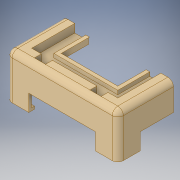
# Autodesk Inventor part: model for case_back
Saved by Autodesk Inventor 2016 (Build 200138000, 138)
## iProperties
Created: 2016-08-06
Part Number: model for case_back
Material: Polyethylene, High Density
Document SubType Name: Modeling
Designer: Jorian Brusind
Density: 0.952 g/cm^3
Appearance: Smooth - Off-White
Author: Jorian Brusind
Autodesk Inventor part; units mm, degrees
ref_plane "YZ Plane" through (0, 0, 0) normal (1, 0, 0) x (0, 1, 0)
ref_plane "XZ Plane" through (0, 0, 0) normal (0, 1, 0) x (-1, 0, 0)
ref_plane "XY Plane" through (0, 0, 0) normal (0, 0, 1) x (1, 0, 0)
sketch "Sketch4" plane through (0, 0, 0) normal (0, 1, 0) x (-1, 0, 0)
  line L0 (0, 0) -> (127, 0)
  line L1 (127, 0) -> (127, -127)
  line L2 (127, -127) -> (0, -127)
  line L3 (0, -127) -> (0, 0)
  dimension "d16" = 127
  dimension "d17" = 127
  constraints: 8 end point, 2 parallel, 1 horizontal, 1 perpendicular
  measures "d16" distance of L1.end L2.end
  measures "d17" distance of L0.end L1.end
extrude "Extrusion4" add sketch "Sketch4" along normal blind 50.8
sketch "Sketch5" plane through (0, 50.8, 0) normal (0, 1, 0) x (1, 0, 0)
  line L0 (0, 0) -> (0, 127) projected
  line L1 (-127, 127) -> (-127, 0) projected
  line L2 (-127, 0) -> (0, 0) projected
  line L3 (0, 127) -> (-127, 127) projected
  line L4 (0, 127) -> (0, 114.3)
  line L5 (-127, 0) -> (-127, 14.2875)
  line L6 (-112.6998, 14.2875) -> (-14.2748, 14.2875)
  line L7 (-14.2748, 14.2875) -> (-14.2748, 112.7125)
  line L8 (-14.2748, 112.7125) -> (-112.6998, 112.7125)
  line L9 (-112.6998, 112.7125) -> (-112.6998, 14.2875)
  line L10 (-112.6998, 14.2875) -> (-112.6998, 26.9875)
  line L11 (-99.9998, 26.9875) -> (-26.9748, 26.9875)
  line L12 (-14.2748, 14.2875) -> (-26.9748, 14.2875)
  line L13 (-26.9748, 26.9875) -> (-26.9748, 100.0125)
  line L14 (-112.6998, 112.7125) -> (-99.9998, 112.7125)
  line L15 (-99.9998, 100.0125) -> (-99.9998, 26.9875)
  line L16 (-112.6998, 112.7125) -> (-112.6998, 100.0125)
  line L17 (-99.9998, 100.0125) -> (-26.9748, 100.0125)
  dimension "d98" = 14.2875
  dimension "d99" = 112.7252
  dimension "d100" = 98.425
  dimension "d101" = 98.425
  dimension "d102" = 12.7
  dimension "d103" = 12.7
  dimension "d104" = 12.7
  dimension "d105" = 12.7
  dimension "d106" = 12.7
  dimension "d107" = 12.7
  dimension "d108" = 12.7
  dimension "d109" = 12.7
  dimension "d110" = 14.3002
  constraints: 28 end point, 8 perpendicular, 6 point on line
  measures "d98" distance of L1.end L5.end
  measures "d99" distance of L5.end L6.end
  measures "d100" distance of L6.end L7.end
  measures "d101" distance of L7.end L8.end
  measures "d102" distance of L6.start L10.end
  measures "d103" distance of L6.end L12.end
  measures "d104" distance of L8.end L14.end
  measures "d105" distance of L8.end L16.end
  measures "d106" distance between parallel lines of L9 L15
  measures "d107" distance between parallel lines of L7 L13
  measures "d108" distance between parallel lines of L8 L17
  measures "d109" distance between parallel lines of L6 L11
  measures "d110" distance between parallel lines of L1 L9
sketch "Sketch13" plane through (0, 50.8, 0) normal (0, 1, 0) x (1, 0, 0)
  line L0 (-127, 127) -> (-127, 0) projected
  line L1 (-127, 0) -> (-88.9, 0)
  line L2 (0, 127) -> (0, 0) projected
  line L3 (0, 0) -> (-38.1, 0)
  line L4 (-127, 0) -> (0, 0) projected
  line L5 (-88.9, 0) -> (-88.9, 14.3002)
  line L6 (-38.1, 0) -> (-38.1, 14.3002)
  line L7 (-88.9, 14.3002) -> (-101.6, 14.3002)
  line L8 (-101.6, 14.3002) -> (-101.6, 6.35)
  line L9 (-101.6, 6.35) -> (-88.9, 6.35)
  line L10 (-88.9, 6.35) -> (-88.9, 14.3002)
  line L11 (-38.1, 14.3002) -> (-25.4, 14.3002)
  line L12 (-25.4, 14.3002) -> (-25.4, 6.35)
  line L13 (-25.4, 6.35) -> (-38.1, 6.35)
  line L14 (-38.1, 6.35) -> (-38.1, 14.3002)
  dimension "d65" = 38.1
  dimension "d66" = 38.1
  dimension "d67" = 12.7
  dimension "d68" = 7.9502
  dimension "d69" = 12.7
  dimension "d70" = 7.9502
  dimension "d113" = 6.35
  dimension "d114" = 6.35
  constraints: 24 end point, 5 parallel, 3 horizontal, 2 perpendicular, 1 point on line, 1 vertical
  measures "d65" distance of L0.end L1.end
  measures "d66" distance of L2.end L3.end
  measures "d67" distance of L9.end L8.end
  measures "d68" distance of L8.end L7.end
  measures "d69" distance of L12.end L13.end
  measures "d70" distance of L11.end L12.end
  measures "d113" distance between parallel lines of L4 L13
  measures "d114" distance between parallel lines of L4 L9
extrude "Extrusion11" cut sketch "Sketch13" against normal blind 25.4
extrude "Extrusion13" cut sketch "Sketch5" against normal blind 9.525 contours L9 L8 L7 L6
chamfer "Chamfer1" distance 4.7625 angle 45 4 edges at (-63.4873, 50.8, -100.0125) (-99.9998, 50.8, -63.5) (-63.4873, 50.8, -26.9875) (-26.9748, 50.8, -63.5)
shell "Shell1" thickness 3.175 removed faces 0
sketch "Sketch16" plane through (0, 0, 0) normal (0, -1, 0) x (1, 0, 0)
  line L0 (-127, 0) -> (0, 0) projected
  line L1 (-127, 0) -> (-101.6, 0)
  line L2 (-88.9, -6.35) -> (-101.6, -6.35) projected
  line L3 (-101.6, 0) -> (-101.6, -6.35)
  line L4 (-101.6, -6.35) -> (-120.65, -6.35)
  line L5 (-120.65, -6.35) -> (-120.65, -25.4)
  line L6 (-120.65, -25.4) -> (-127, -25.4)
  line L7 (-127, -25.4) -> (-127, 0)
  line L8 (0, 0) -> (-25.4, 0)
  line L9 (-25.4, 0) -> (-25.4, -6.35)
  line L10 (-25.4, -6.35) -> (-6.35, -6.35)
  line L11 (-6.35, -6.35) -> (-6.35, -25.4)
  line L12 (-6.35, -25.4) -> (0, -25.4)
  line L13 (0, 0) -> (0, -127) projected
  line L14 (0, -25.4) -> (0, 0)
  line L15 (-127, -127) -> (-127, 0) projected
  line L16 (-127, -127) -> (-101.6, -127)
  line L17 (-101.6, -127) -> (-101.6, -120.65)
  line L18 (-101.6, -120.65) -> (-120.65, -120.65)
  line L19 (-120.65, -120.65) -> (-120.65, -101.6)
  line L20 (-120.65, -101.6) -> (-127, -101.6)
  line L21 (-127, -127) -> (-127, -101.6)
  line L22 (0, -127) -> (-25.4, -127)
  line L23 (-25.4, -127) -> (-25.4, -120.65)
  line L24 (-25.4, -120.65) -> (-6.35, -120.65)
  line L25 (-6.35, -120.65) -> (-6.35, -101.6)
  line L26 (-6.35, -101.6) -> (0, -101.6)
  line L27 (0, -101.6) -> (0, -127)
  line L28 (-127, -127) -> (0, -127)
  line L29 (0, -127) -> (0, 0)
  line L30 (0, 0) -> (-127, 0)
  line L31 (-127, 0) -> (-127, -127)
  dimension "d148" = 25.4
  dimension "d149" = 19.05
  dimension "d150" = 19.05
  dimension "d151" = 25.4
  dimension "d152" = 6.35
  dimension "d153" = 19.05
  dimension "d154" = 19.05
  dimension "d155" = 25.4
  dimension "d156" = 6.35
  dimension "d157" = 19.05
  dimension "d158" = 6.35
  dimension "d159" = 25.4
  dimension "d160" = 6.35
  dimension "d161" = 19.05
  dimension "d162" = 25.4
  constraints: 56 end point, 17 perpendicular, 4 point on line, 3 horizontal, 3 vertical, 2 parallel
  measures "d148" distance of L0.start L1.end
  measures "d149" distance of L2.end L4.end
  measures "d150" distance of L4.end L5.end
  measures "d151" distance of L0.end L8.end
  measures "d152" distance of L8.end L9.end
  measures "d153" distance of L9.end L10.end
  measures "d154" distance of L10.end L11.end
  measures "d155" distance of L15.start L16.end
  measures "d156" distance of L16.end L17.end
  measures "d157" distance of L18.end L19.end
  measures "d158" distance of L19.end L20.end
  measures "d159" distance of L13.end L22.end
  measures "d160" distance of L25.end L26.end
  measures "d161" distance of L24.end L25.end
  measures "d162" distance of L26.end L13.end
extrude "Extrusion15" cut sketch "Sketch16" against normal blind 19.05 contours L0 L9 L10 L11 L12 L13 L26 L25 L24 L23 L28 L17 L18 L19 L20 L15 L6 L5 L4 L3
fillet "Fillet1" radius 6.35 8 edges at (0, 25.4, 0) (0, 25.4, -127) (-127, 25.4, 0) (-127, 25.4, -127) (-127, 50.8, -63.5) (-63.5, 50.8, 0) (-63.5, 50.8, -127) (0, 50.8, -63.5)
sketch "Sketch25" plane through (0, 50.8, 0) normal (0, 1, 0) x (1, 0, 0)
  line L0 (-99.9998, 100.0125) -> (-95.2373, 95.25) projected
  line L1 (-99.9998, 26.9875) -> (-26.9748, 26.9875) projected
  line L2 (-99.9998, 100.0125) -> (-26.9748, 100.0125)
  line L3 (-26.9748, 100.0125) -> (-26.9748, 26.9875)
  line L4 (-26.9748, 26.9875) -> (-99.9998, 26.9875)
  line L5 (-99.9998, 26.9875) -> (-99.9998, 100.0125)
  point P0 (0, 0)
  constraints: 8 end point, 2 parallel, 1 horizontal, 1 perpendicular
extrude "Extrusion24" cut sketch "Sketch25" against normal blind 5.08
sketch "Sketch26" plane through (-115.8748, 38.1, -115.8875) normal (0, -1, 0) x (1, 0, 0)
  line L0 (74.5998, 104.775) -> (30.1498, 104.775) projected
  line L1 (19.05, 85.725) -> (85.725, 85.725) projected
  line L2 (74.5998, 104.775) -> (30.1498, 104.775)
  line L3 (30.1498, 104.775) -> (30.1498, 85.725)
  line L4 (30.1498, 85.725) -> (74.5998, 85.725)
  line L5 (74.5998, 85.725) -> (74.5998, 104.775)
  point P0 (115.8748, 115.8875)
  constraints: 8 end point, 2 parallel, 1 horizontal, 1 perpendicular, 1 point on line
extrude "Extrusion25" add sketch "Sketch26" along normal blind 6.35
sketch "Sketch27" plane through (-85.725, 38.1, -30.1625) normal (-1, 0, 0) x (0, 0, 1)
  line L0 (0, 0) -> (0, -6.35) projected
  line L1 (0, 0) -> (19.05, 0)
  line L2 (19.05, 9.525) -> (19.05, -6.35) projected
  line L3 (0, 0) -> (12.6873, 0) projected
  line L4 (12.6873, -6.35) -> (0, -6.35) projected
  line L5 (0, 0) -> (0, -6.35)
  line L6 (12.6873, -6.35) -> (19.05, -6.35) projected
  line L7 (0, -6.35) -> (19.05, -6.35)
  line L8 (19.05, -6.35) -> (19.05, 0)
  line L9 (0, -6.35) -> (9.525, -6.35)
  line L10 (9.525, -3.175) -> (9.525, -6.35)
  spline S0 degree 2 poles (19.05, -6.35) (9.525, 0) (0, -6.35) knots 0 0 0 1 1 1
  point P0 (30.1625, -38.1)
  constraints: 12 end point, 3 collinear, 1 midpoint, 1 perpendicular, 1 point on line, 1 vertical, 3 other
extrude "Extrusion26" cut sketch "Sketch27" against normal blind 44.45 contours S0 L10 L4 | L10 S0 L6 L4
sketch "Sketch28" plane through (-30.1498, 44.7224, -30.1625) normal (0, 0, -1) x (-1, 0, 0)
  line L0 (55.5752, -6.6224) -> (42.8752, -6.6224)
  line L1 (11.1252, -6.6224) -> (23.8252, -6.6224)
  line L2 (42.8752, -6.6224) -> (39.0652, -6.6224)
  line L3 (39.0652, -6.6224) -> (39.0652, -5.0984)
  line L4 (39.0652, -5.0984) -> (42.8752, -5.0984)
  line L5 (42.8752, -5.0984) -> (42.8752, -6.6224)
  line L6 (23.8252, -6.6224) -> (27.6352, -6.6224)
  line L7 (27.6352, -6.6224) -> (27.6352, -5.0984)
  line L8 (27.6352, -5.0984) -> (23.8252, -5.0984)
  line L9 (23.8252, -5.0984) -> (23.8252, -6.6224)
  point P0 (-30.1498, -44.7224)
  dimension "d226" = 12.7
  dimension "d227" = 12.7
  dimension "d228" = 3.81
  dimension "d229" = 1.524
  dimension "d230" = 3.81
  dimension "d231" = 1.524
  constraints: 20 end point, 4 horizontal, 4 parallel, 2 perpendicular
  measures "d226" distance of L0.start L0.end
  measures "d227" distance of L1.start L1.end
  measures "d228" distance of L3.end L4.end
  measures "d229" distance of L2.end L3.end
  measures "d230" distance of L8.end L7.end
  measures "d231" distance of L7.end L6.end
extrude "Extrusion27" cut sketch "Sketch28" against normal blind 19.05
sketch "Sketch29" plane through (-115.8748, 38.1, -115.8875) normal (0, -1, 0) x (1, 0, 0)
  line L0 (85.725, 85.725) -> (85.725, 19.05) projected
  line L1 (88.9, 88.9) -> (88.9, 15.875) projected
  line L2 (15.875, 15.875) -> (15.875, 88.9) projected
  line L3 (19.05, 19.05) -> (19.05, 85.725) projected
  line L4 (19.05, 85.725) -> (19.05, 34.925)
  line L5 (74.5998, 85.725) -> (85.725, 85.725) projected
  line L6 (85.725, 85.725) -> (85.725, 34.925)
  line L7 (19.05, 34.925) -> (15.875, 34.925)
  line L8 (85.725, 34.925) -> (88.9, 34.925)
  line L9 (112.6998, -7.9375) -> (-7.9502, -7.9375) projected
  line L10 (15.875, 34.925) -> (22.225, 34.925)
  line L11 (22.225, 34.925) -> (22.225, -7.9375)
  line L12 (22.225, -7.9375) -> (15.875, -7.9375)
  line L13 (15.875, -7.9375) -> (15.875, 34.925)
  line L14 (88.9, 34.925) -> (82.55, 34.925)
  line L15 (82.55, 34.925) -> (82.55, -7.9375)
  line L16 (82.55, -7.9375) -> (88.9, -7.9375)
  line L17 (88.9, -7.9375) -> (88.9, 34.925)
  point P0 (115.8748, 115.8875)
  point P1 (88.9, 19.05)
  point P2 (15.875, 19.05)
  dimension "d247" = 50.8
  dimension "d248" = 50.8
  dimension "d249" = 3.175
  dimension "d250" = 3.175
  dimension "d251" = 6.35
  dimension "d252" = 6.35
  constraints: 24 end point, 8 point on line, 4 parallel, 2 horizontal, 2 perpendicular
  measures "d247" distance of L3.end L4.end
  measures "d248" distance of L0.start L6.end
  measures "d249" distance of L4.end L7.end
  measures "d250" distance of L6.end L8.end
  measures "d251" distance of L11.end L12.end
  measures "d252" distance of L16.end L15.end
extrude "Extrusion28" add sketch "Sketch29" along normal blind 4.7625
sketch "Sketch31" plane through (-96.8248, 38.1, -80.9625) normal (0, 0, 1) x (1, 0, 0)
  line L0 (3.175, 0) -> (0, 0)
  line L1 (0, 0) -> (0, -3.175)
  line L2 (0, -3.175) -> (3.175, -3.175)
  line L3 (3.175, -3.175) -> (3.175, 0)
  line L4 (66.675, 0) -> (63.5, 0) projected
  line L5 (63.5, 0) -> (66.675, 0)
  line L6 (66.675, 0) -> (66.675, -3.175)
  line L7 (66.675, -3.175) -> (63.5, -3.175)
  line L8 (63.5, -3.175) -> (63.5, 0)
  point P0 (96.8248, -38.1)
  dimension "d253" = 3.175
  dimension "d254" = 3.175
  dimension "d255" = 3.175
  dimension "d256" = 3.175
  constraints: 16 end point, 4 parallel, 2 horizontal, 2 perpendicular
  measures "d253" distance of L2.end L1.end
  measures "d254" distance of L1.end L0.end
  measures "d255" distance of L6.end L7.end
  measures "d256" distance of L5.end L6.end
extrude "Extrusion30" cut sketch "Sketch31" against normal blind 42.8752
sketch "Sketch33" plane through (0, 0, -25.4) normal (1, 0, 0) x (0, 0, -1)
  line L0 (-25.4, 0) -> (38.1, 0)
  line L1 (38.1, 0) -> (38.1, 50.8)
  line L2 (-11.1125, 50.8) -> (87.3125, 50.8) projected
  dimension "d259" = 63.5
  constraints: 4 end point, 1 horizontal, 1 midpoint
  measures "d259" distance of L0.start L0.end
split body "Split2" sketch "Sketch33" result one side removed curves L0 L1 removed pieces at (-73.5499, 44.45, -124.325)
body "Solid2"
